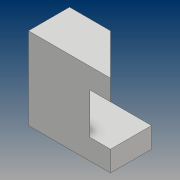
# Autodesk Inventor part: 48 (22000.000 mm^3)
Saved by Autodesk Inventor 2018 (Build 220112000, 112)
## iProperties
Created: 2020-09-18
Part Number: 48 (22000.000 mm^3)
Material: 一般
Document SubType Name: Modeling
Designer: 88697
Density: 1 g/cm^3
Appearance: 預設
Author: 88697
Autodesk Inventor part; units mm, degrees
ref_plane "YZ Plane" through (0, 0, 0) normal (1, 0, 0) x (0, 1, 0)
ref_plane "XZ Plane" through (0, 0, 0) normal (0, 1, 0) x (-1, 0, 0)
ref_plane "XY Plane" through (0, 0, 0) normal (0, 0, 1) x (1, 0, 0)
sketch "草圖1" plane through (0, 0, 0) normal (0, 0, 1) x (1, 0, 0)
  line L0 (0, 0) -> (40, 0)
  line L1 (40, 0) -> (40, 20)
  line L2 (40, 20) -> (0, 20)
  line L3 (0, 20) -> (0, 0)
  dimension "d0" = 40
  dimension "d1" = 20
  constraints: 8 end point, 2 parallel, 1 horizontal, 1 perpendicular
  measures "d0" distance of L0.start L0.end
  measures "d1" distance of L2.end L0.start
extrude "擠出1" add sketch "草圖1" along normal blind 10
sketch "草圖2" plane through (0, 0, 10) normal (0, 0, 1) x (1, 0, 0)
  line L0 (40, 20) -> (0, 20) construction
  line L1 (10, 20) -> (30, 0)
  line L2 (0, 0) -> (40, 0) construction
  line L3 (0, 0) -> (40, 0) projected
  line L4 (40, 0) -> (40, 20) projected
  line L5 (40, 20) -> (0, 20) projected
  line L6 (0, 20) -> (0, 0) projected
  line L7 (30, 0) -> (-0.2906, 0)
  line L8 (0, 20) -> (10, 20)
  dimension "d4" = 10
  dimension "d5" = 30
  constraints: 6 end point, 6 point on line
  measures "d4" distance from line of L1.start L6
  measures "d5" distance of L2.start L1.end
extrude "擠出2" add sketch "草圖2" along normal blind 20 contours L1 L3 L6 L5
sketch "草圖3" plane through (0, 0, 30) normal (0, 0, 1) x (1, 0, 0)
  line L0 (0, 0) -> (0, 20)
  line L1 (0, 20) -> (20, 20)
  line L2 (40, 20) -> (0, 20) projected
  line L3 (0, 0) -> (40, 0) projected
  line L4 (40, 0) -> (20, 20)
  line L5 (0, 0) -> (40, 0)
  line L6 (40, 0) -> (40, 20) projected
  dimension "d8" = 20
  constraints: 8 end point, 1 collinear, 1 midpoint, 1 vertical
  measures "d8" distance from line of L6 L1.end
extrude "擠出3" add sketch "草圖3" along normal blind 10 contours L0 L1 L4 L3
